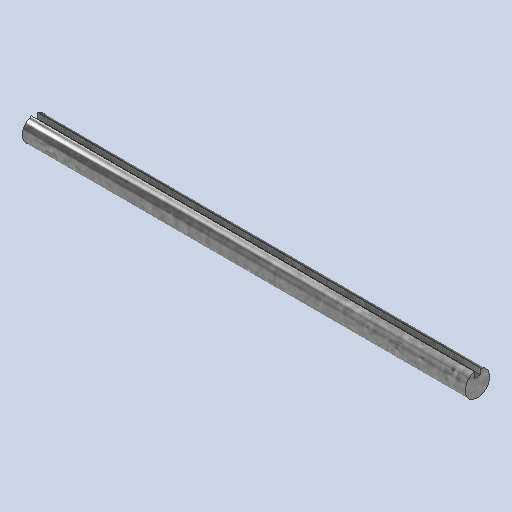
# Autodesk Inventor part: SteelDeadAxel
Saved by Autodesk Inventor 2023 (Build 270158000, 158)
## iProperties
Created: 2022-09-11
Part Number: SteelDeadAxel
Material: Generic
Document SubType Name: Modeling
Designer: PC
Density: 1 g/cm^3
Appearance: Default
Author: PC
Autodesk Inventor part; units mm, degrees
ref_plane "YZ Plane" through (0, 0, 0) normal (1, 0, 0) x (0, 1, 0)
ref_plane "XZ Plane" through (0, 0, 0) normal (0, 1, 0) x (-1, 0, 0)
ref_plane "XY Plane" through (0, 0, 0) normal (0, 0, 1) x (1, 0, 0)
sketch "Sketch1" plane through (0, 0, 0) normal (1, 0, 0) x (0, 1, 0)
  circle A0 centre (0, 0) radius 6.35
  line L0 (9.525, 1.5875) -> (3.175, 1.5875)
  line L1 (3.175, 1.5875) -> (3.175, -1.5875)
  line L2 (3.175, -1.5875) -> (9.525, -1.5875)
  line L3 (9.525, -1.5875) -> (9.525, 1.5875)
  line L4 (9.525, 1.5875) -> (3.175, -1.5875) construction
  line L5 (3.175, 1.5875) -> (9.525, -1.5875) construction
  point P0 (6.35, 0)
  point P1 (6.1484, 1.5875)
  point P2 (6.1484, -1.5875)
  dimension "d0" = 12.7
  dimension "d1" = 3.175
  dimension "d2" = 6.35
  constraints: 12 end point, 2 midpoint, 2 parallel, 1 coincident, 1 horizontal, 1 perpendicular, 3 other
  measures "d1" distance of L0.end L1.end
  measures "d2" distance of L1.end L2.end
extrude "Extrusion1" add sketch "Sketch1" along normal blind 228.6 contours L0 L1 L2 A0 picked at (0, 0)
body "Solid1"
